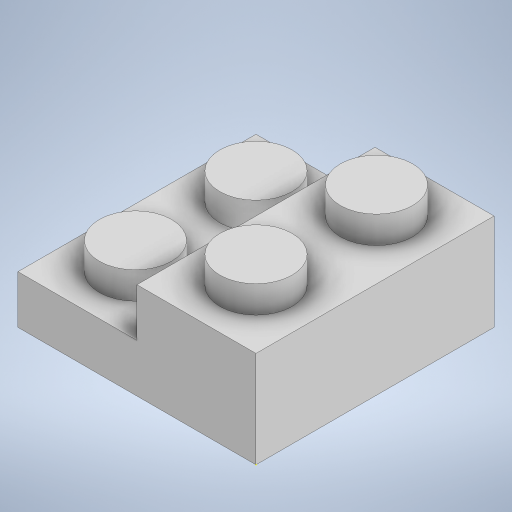
# Autodesk Inventor part: LEGO_hanging_brick
Saved by Autodesk Inventor 2024 (Build 280153000, 153)
## iProperties
Created: 2024-01-05
Part Number: LEGO_hanging_brick
Material: Generic
Document SubType Name: Modeling
Designer: kamil
Density: 1 g/cm^3
Appearance: Default
Author: kamil
Autodesk Inventor part; units mm, degrees
ref_plane "YZ Plane" through (0, 0, 0) normal (1, 0, 0) x (0, 1, 0)
ref_plane "XZ Plane" through (0, 0, 0) normal (0, 1, 0) x (-1, 0, 0)
ref_plane "XY Plane" through (0, 0, 0) normal (0, 0, 1) x (1, 0, 0)
sketch "Sketch1" plane through (0, 0, 0) normal (0, 1, 0) x (-1, 0, 0)
  line L0 (0, 0) -> (15.8, 0)
  line L1 (15.8, 0) -> (15.8, -15.8)
  line L2 (15.8, -15.8) -> (0, -15.8)
  line L3 (0, -15.8) -> (0, 0)
  dimension "d0" = 15.8
  dimension "d1" = 15.8
  constraints: 8 end point, 2 parallel, 1 horizontal, 1 perpendicular
  measures "d0" distance of L1.end L2.end
  measures "d1" distance of L0.end L1.end
extrude "Extrusion1" add sketch "Sketch1" along normal blind 3.2
sketch "Sketch2" plane through (0, 3.2, 0) normal (0, 1, 0) x (1, 0, 0)
  line L0 (-15.8, 0) -> (0, 0) projected
  line L1 (0, 15.8) -> (-15.8, 15.8) projected
  line L2 (0, 0) -> (-7.9, 0)
  line L3 (-7.9, 0) -> (-7.9, 15.8)
  line L4 (-7.9, 15.8) -> (0, 15.8)
  line L5 (0, 15.8) -> (0, 0)
  dimension "d4" = 7.9
  constraints: 8 end point, 2 parallel, 1 horizontal, 1 midpoint, 1 perpendicular
  measures "d4" distance of L3.end L4.end
extrude "Extrusion2" add sketch "Sketch2" along normal blind 3.2
sketch "Sketch3" plane through (0, 6.4, 0) normal (0, 1, 0) x (1, 0, 0)
  circle A0 centre (-3.9, 11.9) radius 2.4
  line L0 (0, 15.8) -> (-7.9, 15.8) projected
  line L1 (0, 0) -> (0, 15.8) projected
  line L2 (0, 7.9) -> (-7.9, 7.9) construction
  line L3 (-7.9, 15.8) -> (-7.9, 0) construction
  circle A1 centre (-3.9, 3.9) radius 2.4
  dimension "d7" = 4.8
  dimension "d8" = 3.9
  dimension "d9" = 3.9
  dimension "d10" = 8
  constraints: 2 centre point, 2 end point, 2 midpoint, 1 symmetric about line, 1 other
  measures "d7" diameter of A0
  measures "d8" distance from line of L0 A0.centre
  measures "d9" distance from line of L1 A0.centre
  measures "d10" distance of A1.centre A0.centre
sketch "Sketch4" plane through (0, 3.2, 0) normal (0, 1, 0) x (1, 0, 0)
  circle A0 centre (-11.9, 11.9) radius 2.4
  line L0 (-7.9, 15.8) -> (-15.8, 15.8) projected
  line L1 (-15.8, 15.8) -> (-15.8, 0) projected
  line L2 (-7.9, 15.8) -> (-7.9, 0) construction
  line L3 (-7.9, 7.9) -> (-15.8, 7.9) construction
  circle A1 centre (-11.9, 3.9) radius 2.4
  point P0 (0, 0)
  dimension "d11" = 4.8
  dimension "d12" = 3.9
  dimension "d13" = 3.9
  constraints: 2 centre point, 2 end point, 2 midpoint, 1 symmetric about line, 1 other
  measures "d11" diameter of A0
  measures "d12" distance from line of L0 A0.centre
  measures "d13" distance from line of L1 A0.centre
extrude "Extrusion3" add sketch "Sketch4" along normal blind 1.8
extrude "Extrusion4" add sketch "Sketch3" along normal blind 1.8
sketch "Sketch5" plane through (0, 0, 0) normal (0, -1, 0) x (1, 0, 0)
  point P0 (0, 0)
body "Solid1"
